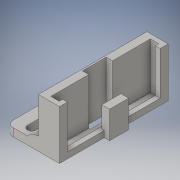
# Autodesk Inventor part: better ultrasonic holder
Saved by Autodesk Inventor 2016 (Build 200138000, 138)
## iProperties
Created: 2017-09-28
Part Number: better ultrasonic holder
Material: Generic
Document SubType Name: Modeling
Designer: T-money
Density: 1 g/cm^3
Appearance: Default
Author: T-money
Autodesk Inventor part; units mm, degrees
ref_plane "YZ Plane" through (0, 0, 0) normal (1, 0, 0) x (0, 1, 0)
ref_plane "XZ Plane" through (0, 0, 0) normal (0, 1, 0) x (-1, 0, 0)
ref_plane "XY Plane" through (0, 0, 0) normal (0, 0, 1) x (1, 0, 0)
sketch "Sketch1" plane through (0, 0, 0) normal (0, 1, 0) x (-1, 0, 0)
  line L0 (0, 0) -> (2.032, 0) construction
  line L1 (0, 0) -> (-2.032, 0) construction
  line L2 (-4.318, 0) -> (-4.318, 3.81)
  line L3 (-4.318, 3.81) -> (5.842, 3.81)
  line L4 (-2.032, 0) -> (-2.032, 1.651)
  line L5 (-2.032, 1.651) -> (2.032, 1.651)
  line L6 (2.032, -46.228) -> (-2.032, -46.228)
  line L7 (-2.032, -46.228) -> (-2.032, -44.577)
  line L8 (-4.318, -44.577) -> (-4.318, -48.387)
  line L9 (-4.318, -48.387) -> (5.842, -48.387)
  line L10 (2.032, 1.651) -> (2.032, -16.5735)
  line L11 (2.032, -16.5735) -> (4.572, -16.5735)
  line L12 (4.572, -16.5735) -> (4.572, -28.0035)
  line L13 (4.572, -28.0035) -> (2.032, -28.0035)
  line L14 (2.032, -28.0035) -> (2.032, -46.228)
  line L15 (5.842, 3.81) -> (5.842, -48.387)
  line L16 (-2.032, -40.8058) -> (4.191, -40.8058) construction
  line L17 (-2.032, 0) -> (-2.032, -44.577)
  line L18 (-4.318, 0) -> (-4.318, -44.577)
  dimension "d0" = 2.032
  dimension "d1" = 2.032
  dimension "d3" = 2.286
  dimension "d5" = 3.81
  dimension "d7" = 10.16
  dimension "d8" = 4.064
  dimension "d9" = 2.159
  dimension "d10" = 1.651
  dimension "d12" = 2.286
  dimension "d13" = 3.81
  dimension "d14" = 1.651
  dimension "d15" = 4.064
  dimension "d16" = 10.16
  dimension "d17" = 11.43
  dimension "d18" = 2.159
  dimension "d19" = 18.2245
  dimension "d21" = 6.223
  dimension "d22" = 2.54
  dimension "d37" = 18.2245
  dimension "d38" = 52.197
  dimension "d39" = 44.577
  constraints: 38 end point, 6 horizontal, 5 perpendicular, 5 vertical, 2 point on line, 1 parallel
  measures "d0" distance of L0.start L0.end
  measures "d1" distance of L0.start L1.end
  measures "d3" distance of L1.end L2.start
  measures "d5" distance of L2.start L2.end
  measures "d7" distance of L2.end L3.end
  measures "d8" distance of L4.end L5.end
  measures "d9" distance between parallel lines of L3 L5
  measures "d10" distance of L1.end L4.end
  measures "d12" distance of L7.end L8.start
  measures "d13" distance of L8.start L8.end
  measures "d14" distance of L6.end L7.end
  measures "d15" distance of L6.start L6.end
  measures "d16" distance of L8.end L9.end
  measures "d17" distance of L11.end L12.end
  measures "d18" distance between parallel lines of L9 L6
  measures "d19" distance of L13.end L6.start
  measures "d21" distance of L16.start L16.end
  measures "d22" distance of L12.end L13.end
  measures "d37" distance of L5.end L10.end
  measures "d38" distance of L3.end L9.end
  measures "d39" distance of L2.start L8.start
extrude "Extrusion1" add sketch "Sketch1" along normal blind 2.9845
sketch "Sketch10" plane through (0, 0, 0) normal (0, -1, 0) x (1, 0, 0)
  line L0 (-2.032, 1.651) -> (-2.032, -16.5735) projected
  line L1 (2.032, -46.228) -> (2.032, 1.651) projected
  line L2 (-2.032, 1.651) -> (2.032, 1.651)
  line L3 (2.032, 1.651) -> (2.032, -46.228)
  line L4 (2.032, -46.228) -> (-2.032, -46.228)
  line L5 (-2.032, -46.228) -> (-2.032, 1.651)
  point P0 (0, 0)
  constraints: 8 end point, 2 parallel, 1 horizontal, 1 perpendicular
extrude "Extrusion5" add sketch "Sketch10" against normal blind 1.27
sketch "Sketch11" plane through (0, 2.9845, 0) normal (0, 1, 0) x (1, 0, 0)
  line L0 (4.318, -3.81) -> (-5.842, -3.81)
  line L1 (-5.842, -3.81) -> (-5.842, 48.387) projected
  line L2 (-5.842, -3.81) -> (-5.842, 48.387)
  line L3 (4.318, 48.387) -> (4.318, 44.577) construction
  line L4 (4.318, -3.81) -> (4.318, 48.387) construction
  line L5 (4.318, -3.81) -> (4.318, 0) construction
  line L6 (4.318, -3.81) -> (4.318, 0)
  line L7 (4.318, 0) -> (2.032, 0)
  line L8 (2.032, 46.228) -> (2.032, -1.651) projected
  line L9 (2.032, -1.651) -> (-2.032, -1.651) projected
  line L10 (2.032, -1.651) -> (-2.032, -1.651)
  line L11 (-2.032, 28.0035) -> (-2.032, 16.5735) projected
  line L12 (-2.032, -1.651) -> (-2.032, 16.5735)
  line L13 (-2.032, -1.651) -> (-2.032, 16.5735) projected
  line L14 (-4.572, 16.5735) -> (-2.032, 16.5735) projected
  line L15 (-2.032, 16.5735) -> (-4.572, 16.5735)
  line L16 (-4.572, 16.5735) -> (-4.572, 28.0035) projected
  line L17 (-4.572, 16.5735) -> (-4.572, 28.0035)
  line L18 (-2.032, 28.0035) -> (-4.572, 28.0035) projected
  line L19 (-4.572, 28.0035) -> (-2.032, 28.0035)
  line L20 (-2.032, 28.0035) -> (-2.032, 46.228)
  line L21 (-2.032, 46.228) -> (2.032, 46.228)
  line L22 (2.032, 46.228) -> (2.032, 44.577)
  line L23 (2.032, 44.577) -> (4.318, 44.577)
  line L24 (4.318, 44.577) -> (4.318, 48.387)
  line L25 (-5.842, 48.387) -> (4.318, 48.387)
  point P0 (0, 0)
  dimension "d43" = 3.81
  dimension "d44" = 3.81
  constraints: 34 end point, 6 collinear, 5 point on line, 4 horizontal, 3 perpendicular
  measures "d43" distance of L3.start L3.end
  measures "d44" distance of L0.start L5.end
extrude "Extrusion6" add sketch "Sketch11" along normal blind 20.701 contours L0 L1 L25 L24 L23 L8 L21 L20 L18 L16 L14 L12 L9 L7 L6
sketch "Sketch12" plane through (-5.842, 0, 3.81) normal (0, 0, 1) x (1, 0, 0)
  line L0 (0, 0) -> (0, 23.6855) construction
  line L1 (10.16, 0) -> (0, 0) construction
  line L2 (0, 0) -> (0, 23.6855) projected
  line L3 (0, 0) -> (-6.35, 0) construction
  line L4 (0, 0) -> (0, 6.35) construction
  arc A0 (0, 6.35) -> (-6.35, 0) centre (0, 0) ccw
  line L5 (-6.35, 0) -> (0, 0)
  line L6 (0, 0) -> (0, 6.35)
  point P0 (5.842, 0)
  dimension "d54" = 6.35
  dimension "d55" = 6.35
  dimension "d56" = 6.35
  constraints: 8 end point, 2 point on circle, 1 centre point, 1 horizontal, 1 point on line
  measures "d54" distance of L0.start L3.end
  measures "d55" distance of L0.start L4.end
  measures "d56" radius of A0
extrude "Extrusion7" add sketch "Sketch12" against normal blind 10.16
sketch "Sketch14" plane through (4.318, 0, -48.387) normal (0, 0, -1) x (-1, 0, 0)
  line L0 (10.16, 0) -> (0, 0) projected
  line L1 (10.16, 0) -> (10.16, 6.3521)
  line L2 (10.16, 0) -> (10.16, 23.6855) projected
  line L3 (0, 0) -> (16.51, 0) projected
  line L4 (10.16, 0) -> (16.51, 0)
  arc A0 (16.51, 0) -> (10.16, 6.3521) centre (10.1572, -0.0008) ccw
  point P0 (4.318, 0)
  constraints: 4 end point, 2 point on circle, 1 centre point, 1 horizontal, 1 point on line
extrude "Extrusion8" add sketch "Sketch14" against normal blind 10.16
sketch "Sketch16" plane through (0, 0, 0) normal (0, -1, 0) x (1, 0, 0)
  line L0 (-12.192, -38.227) -> (-5.842, -38.227) projected
  line L1 (-5.842, -38.227) -> (-21.082, -38.227)
  line L2 (-21.082, -38.227) -> (-21.082, -6.35)
  line L3 (-21.082, -6.35) -> (-5.842, -6.35)
  line L4 (-5.842, -6.35) -> (-5.842, -38.227)
  point P0 (0, 0)
  point P1 (-12.192, -6.35)
  dimension "d63" = 15.24
  constraints: 8 end point, 2 parallel, 1 horizontal, 1 perpendicular
  measures "d63" distance of L0.end L1.end
extrude "Extrusion9" add sketch "Sketch16" against normal blind 3.81
sketch "Sketch17" plane through (0, 3.81, 0) normal (0, 1, 0) x (1, 0, 0)
  circle A0 centre (-13.462, 29.4323) radius 1.9844
  circle A1 centre (-13.2021, 15.1448) radius 1.9844
  line L0 (-5.842, 38.227) -> (-5.842, 6.35) construction
  line L1 (-5.842, 36.0862) -> (-21.082, 36.0862) construction
  line L2 (-21.082, 38.227) -> (-21.082, 6.35) construction
  line L3 (-21.082, 37.0641) -> (-13.462, 37.0641) construction
  line L4 (-10.9221, 38.227) -> (-21.082, 38.227) construction
  line L5 (-12.933, 38.227) -> (-12.933, 6.35) construction
  line L6 (-21.082, 6.35) -> (-12.192, 6.35) construction
  line L7 (-21.082, 6.35) -> (-10.922, 6.35) construction
  line L8 (-5.842, 6.35) -> (-10.922, 6.35) construction
  line L9 (-13.462, 29.4323) -> (-13.462, 38.227) construction
  line L10 (-13.2021, 15.1448) -> (-13.2021, 6.35) construction
  point P0 (0, 0)
  dimension "d66" = 3.9688
  dimension "d67" = 3.9688
  dimension "d68" = 15.24
  dimension "d69" = 7.62
  dimension "d70" = 31.877
  dimension "d72" = 7.62
  dimension "d90" = 14.2875
  constraints: 10 end point, 7 point on line, 2 centre point, 2 perpendicular, 2 vertical, 1 horizontal, 1 parallel
  measures "d66" diameter of A0
  measures "d67" diameter of A1
  measures "d68" distance of L1.start L1.end
  measures "d69" distance of L3.start L3.end
  measures "d70" distance of L5.start L5.end
  measures "d72" distance from line of L2 L9.start
  measures "d90" vertical distance of L10.start L9.start
extrude "Extrusion10" cut sketch "Sketch17" against normal blind 3.81
sketch "Sketch18" plane through (4.318, 0, 3.81) normal (1, 0, 0) x (0, 0, -1)
  line L0 (0, 1.944) -> (52.197, 1.944) construction
  line L1 (52.197, 0) -> (52.197, 6.3521) construction
  line L2 (0, 0) -> (0, 23.6855) construction
  line L3 (0, 2.5647) -> (21.5265, 2.5647) construction
  line L4 (48.387, 2.9845) -> (3.81, 2.9845) projected
  line L5 (21.5265, 2.9845) -> (30.6705, 2.9845)
  line L6 (21.5265, 2.9845) -> (21.5265, 13.1445)
  line L7 (21.5265, 13.1445) -> (30.6705, 13.1445)
  line L8 (30.6705, 13.1445) -> (30.6705, 2.9845)
  point P0 (3.81, 0)
  dimension "d79" = 52.197
  dimension "d80" = 21.5265
  dimension "d82" = 10.16
  constraints: 12 end point, 4 point on line, 2 perpendicular, 1 horizontal, 1 parallel, 1 vertical
  measures "d79" distance of L0.start L0.end
  measures "d80" distance of L3.start L3.end
  measures "d82" distance of L5.start L6.end
extrude "Extrusion11" add sketch "Sketch18" against normal blind 2.286
sketch "Sketch20" plane through (0, 23.6855, 0) normal (0, 1, 0) x (1, 0, 0)
  line L0 (-4.572, 16.5735) -> (-4.572, 28.0035) projected
  line L1 (-4.572, 28.0035) -> (-5.0647, 28.0035)
  line L2 (-5.0647, 28.0035) -> (-5.0647, 16.5735)
  line L3 (-5.0647, 16.5735) -> (-4.572, 16.5735)
  line L4 (-4.572, 16.5735) -> (-4.572, 28.0035)
  point P0 (0, 0)
  constraints: 8 end point, 2 parallel, 1 horizontal, 1 perpendicular
extrude "Extrusion12" cut sketch "Sketch20" against normal up to next
sketch "Sketch21" plane through (0, 1.27, 0) normal (0, 1, 0) x (1, 0, 0)
  line L0 (-2.032, 16.5735) -> (-1.2835, 16.5735)
  line L1 (-1.2835, 16.5735) -> (-1.2835, 27.9949)
  line L2 (-1.2835, 27.9949) -> (-2.032, 27.9949)
  line L3 (-2.032, 27.9949) -> (-2.032, 16.5735)
  point P0 (0, 0)
  constraints: 8 end point, 2 parallel, 1 horizontal, 1 perpendicular
extrude "Extrusion13" cut sketch "Sketch21" against normal up to next
sketch "Sketch22" plane through (0, 0, 0) normal (0, -1, 0) x (1, 0, 0)
  line L0 (2.032, -26.8605) -> (4.318, -26.8605) projected
  line L1 (4.318, -26.8605) -> (4.318, -17.6876)
  line L2 (4.318, -48.387) -> (4.318, 3.81) projected
  line L3 (4.318, -26.8605) -> (6.858, -26.8605)
  line L4 (6.858, -26.8605) -> (6.858, -17.7165)
  line L5 (6.858, -17.7165) -> (4.318, -17.7165)
  line L6 (4.318, -17.7165) -> (4.318, -26.8605)
  point P0 (0, 0)
  dimension "d91" = 2.54
  constraints: 10 end point, 2 parallel, 1 horizontal, 1 perpendicular, 1 point on line
  measures "d91" distance of L5.end L4.end
extrude "Extrusion14" add sketch "Sketch22" against normal up to surface (13.1445 mm away)
sketch "Sketch23" plane through (2.032, 13.1445, -17.7165) normal (0, 1, 0) x (1, 0, 0)
  line L0 (0, 9.144) -> (4.826, 9.144) projected
  line L1 (2.286, 0) -> (0, 0) projected
  line L2 (0, 9.144) -> (1.143, 9.144)
  line L3 (1.143, 9.144) -> (1.143, 0)
  line L4 (1.143, 0) -> (0, 0)
  line L5 (0, 0) -> (0, 9.144)
  point P0 (-2.032, -17.7165)
  constraints: 8 end point, 2 parallel, 1 horizontal, 1 midpoint, 1 perpendicular
extrude "Extrusion15" cut sketch "Sketch23" against normal up to surface (10.16 mm away)
sketch "Sketch24" plane through (-5.842, 23.6855, 3.81) normal (0, 0, 1) x (1, 0, 0)
  line L0 (0, -17.3334) -> (0, 0) projected
  line L1 (-6.35, -23.6855) -> (-15.24, -23.6855) projected
  line L2 (-15.24, -23.6855) -> (0, -23.6855)
  line L3 (-15.24, -23.6855) -> (-15.24, -19.8755) projected
  line L4 (-15.24, -23.6855) -> (-15.24, -19.8755)
  line L5 (-5.0801, -19.8755) -> (0, -19.8755) projected
  line L6 (-15.24, -19.8755) -> (0, -19.8755)
  line L7 (0, -19.8755) -> (0, -23.6855)
  point P0 (5.842, -23.6855)
  constraints: 8 end point, 2 collinear, 1 perpendicular
sketch "Sketch25" plane through (0, 3.81, 0) normal (0, 1, 0) x (1, 0, 0)
  line L0 (-15.4123, 29.8338) -> (-11.4776, 29.4323) construction
  circle A0 centre (-13.462, 29.4323) radius 1.9844 construction
  line L1 (-15.4464, 29.4323) -> (-11.4776, 29.4323) construction
  circle A1 centre (-13.462, 29.4323) radius 1.9844 construction
  point P0 (0, 0)
  constraints: 4 end point, 2 point on circle, 1 centre point, 1 coincident, 1 concentric, 1 horizontal
extrude "Extrusion16" add sketch "Sketch24" against normal up to surface (52.197 mm away)
sketch "Sketch26" plane through (0, 3.81, 0) normal (0, 1, 0) x (1, 0, 0)
  line L0 (-13.4927, 29.4297) -> (-13.4927, 21.7166) construction
  line L1 (6.858, 26.8605) -> (6.858, 17.7165) construction
  line L2 (6.858, 22.1055) -> (-21.082, 22.1055) construction
  line L3 (-21.082, -3.81) -> (-21.082, 48.387) construction
  line L4 (-13.4927, 0.6164) -> (-13.4927, 43.5947) construction
  line L5 (-11.4607, 0.6164) -> (-11.4607, 43.5947) construction
  line L6 (-15.5247, 43.5947) -> (-15.5247, 0.6164) construction
  arc A0 (-15.5247, 0.6164) -> (-11.4607, 0.6164) centre (-13.4927, 0.6164) ccw construction
  arc A1 (-11.4607, 43.5947) -> (-15.5247, 43.5947) centre (-13.4927, 43.5947) ccw construction
  line L7 (-13.4927, 0.6164) -> (-13.4927, 43.5947) construction
  line L8 (-11.4607, 0.6164) -> (-11.4607, 43.5947)
  line L9 (-15.5247, 43.5947) -> (-15.5247, 0.6164)
  arc A2 (-15.5247, 0.6164) -> (-11.4607, 0.6164) centre (-13.4927, 0.6164) ccw
  arc A3 (-11.4607, 43.5947) -> (-15.5247, 43.5947) centre (-13.4927, 43.5947) ccw
  point P0 (0, 0)
  point P1 (-13.4927, 22.1055)
  dimension "d98" = 4.064
  constraints: 20 end point, 8 point on circle, 8 tangent, 5 point on line, 4 centre point, 3 equal length, 2 midpoint, 1 concentric, 1 horizontal, 1 vertical
  measures "d98" diameter of A1
extrude "Extrusion17" cut sketch "Sketch26" against normal up to next
fillet "Fillet1" radius 3.175 2 edges at (-21.082, 1.905, 3.81) (-21.082, 1.905, -48.387)
body "Solid1"
